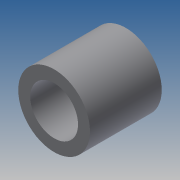
# Autodesk Inventor part: .75in Spacer
Saved by Autodesk Inventor 2014 SP1 (Build 180222100, 222)
## iProperties
Created: 2014-02-01
Part Number: .75in Spacer
Material: Generic
Document SubType Name: Modeling
Designer: Pradhan alexander
Density: 1 g/cm^3
Appearance: Default
Author: Pradhan alexander
Autodesk Inventor part; units mm, degrees
ref_plane "YZ Plane" through (0, 0, 0) normal (1, 0, 0) x (0, 1, 0)
ref_plane "XZ Plane" through (0, 0, 0) normal (0, 1, 0) x (-1, 0, 0)
ref_plane "XY Plane" through (0, 0, 0) normal (0, 0, 1) x (1, 0, 0)
sketch "Sketch1" plane through (0, 0, 0) normal (0, 0, 1) x (1, 0, 0)
  circle A0 centre (-1.2402, 1.3288) radius 6.35
  circle A1 centre (-1.2402, 1.3288) radius 9.525
  dimension "d0" = 12.7
  dimension "d1" = 3.175
  constraints: 2 centre point, 1 coincident
  measures "d0" diameter of A0
  measures "d1" radial gap between concentric circles of A0 A1
extrude "Extrusion1" add sketch "Sketch1" against normal blind 19.05
body "Solid1"
